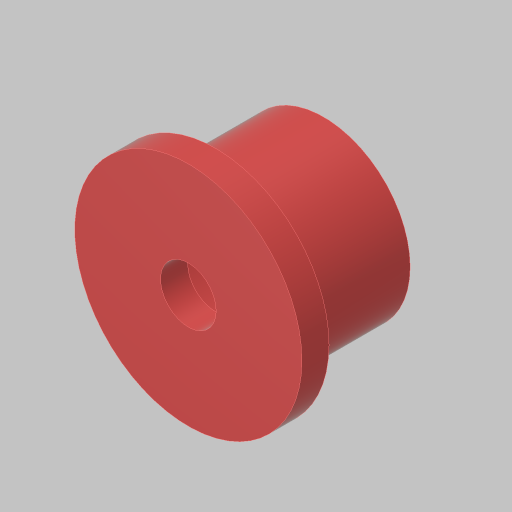
# Autodesk Inventor part: EL2-015
Saved by Autodesk Inventor 2023.5 (Build 275446000, 446)
## iProperties
Created: 2025-01-21
Part Number: EL2-015
Material: ABS Plastic
Document SubType Name: Modeling
Designer: slick
Density: 1.06 g/cm^3
Appearance: Smooth - Red
Author: slick
Autodesk Inventor part; units mm, degrees
ref_plane "YZ Plane" through (0, 0, 0) normal (1, 0, 0) x (0, 1, 0)
ref_plane "XZ Plane" through (0, 0, 0) normal (0, 1, 0) x (-1, 0, 0)
ref_plane "XY Plane" through (0, 0, 0) normal (0, 0, 1) x (1, 0, 0)
sketch "Sketch1" plane through (0, 0, 0) normal (0, 0, 1) x (1, 0, 0)
  circle A0 centre (0, 0) radius 10.16
  circle A1 centre (0, 0) radius 8.7376
  dimension "d0" = 20.32
  dimension "d6" = 17.4752
  constraints: 2 centre point, 2 coincident
  measures "d0" diameter of A0
  measures "d6" diameter of A1
extrude "Extrusion1" add sketch "Sketch1" along normal blind 12.7
sketch "Sketch2" plane through (0, 0, 12.7) normal (0, 0, 1) x (1, 0, 0)
  circle A0 centre (0, 0) radius 10.16 projected
  circle A1 centre (0, 0) radius 13.335
  circle A2 centre (0, 0) radius 8.7376 projected
  dimension "d3" = 3.175
  constraints: 1 centre point
  measures "d3" radial gap between concentric circles of A0 A1
extrude "Extrusion2" add sketch "Sketch2" along normal blind 3.175 contours A0 | A1 | A2
sketch "Sketch3" plane through (0, 0, 15.875) normal (0, 0, 1) x (1, 0, 0)
  point P0 (0, 0)
hole "Hole1" at (0, 0, 15.875) direction (0, 0, -1) diameter 6.5278 end through all clearance for "Flat Head Machine Screw (82)" size "1/4" standard "Ansi Unified Screw Threads"
body "Solid1"
